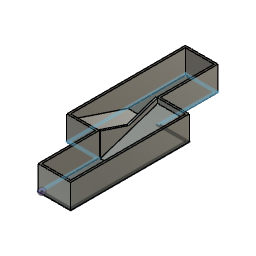
SandGravelMulch v1 (Autodesk Fusion 360 design; units mm, degrees)
Autodesk Fusion 360 part; units mm, degrees
sketch "Sketch1" plane through (0, 0, 0) normal (0, 0, 1) x (1, 0, 0)
  line L0 (0, 0) -> (300, 0)
  line L1 (300, 0) -> (300, 1200)
  line L2 (300, 1200) -> (0, 1200)
  line L3 (0, 600) -> (-300, 600)
  line L4 (-300, 600) -> (-300, 1800)
  line L5 (-300, 1800) -> (0, 1800)
  line L6 (0, 1800) -> (0, 1200)
  line L7 (0, 0) -> (0, 600)
  line L8 (20, 1820) -> (20, 1220)
  line L9 (320, 1220) -> (20, 1220)
  line L10 (320, -20) -> (320, 1220)
  line L11 (-20, -20) -> (320, -20)
  line L12 (-20, -20) -> (-20, 580)
  line L13 (-20, 580) -> (-320, 580)
  line L14 (-320, 580) -> (-320, 1820)
  line L15 (-320, 1820) -> (20, 1820)
  dimension "d1" = 300
  dimension "d2" = 1200
  dimension "d3" = 300
  dimension "d4" = 1200
  dimension "d5" = -20
  constraint horizontal L0
  constraint vertical L1
  constraint horizontal L2
  constraint coincident L0.start L7.start
  constraint perpendicular L3 L4
  constraint perpendicular L4 L5
  constraint perpendicular L2 L6
  constraint perpendicular L3 L7
  measures "d1" distance of L0.start L0.end
  measures "d2" distance of L0.end L1.end
  measures "d3" distance of L3.start L3.end
  measures "d4" distance of L3.end L4.end
extrude "Extrude1" add sketch "Sketch1" along normal blind 400 makes body 1
extrude "Extrude2" add sketch "Sketch1" against normal blind 5 separate body contours L0 L1 L2 L3 L4 L5 L6 L7 makes body 2
extrude "Extrude3" add sketch "Sketch1" against normal blind 5 bodies 1 2
extrude "Extrude4" cut 1 faces at (-313.3333, 1400, 400) along direction (0, 0, -1) blind 100 on bodies 1 bodies 1
extrude "Extrude5" cut 1 faces at (-313.3333, 1400, 300) along direction (0, 0, -1) blind 50 on bodies 1 bodies 1
sketch "Sketch2" plane through (300, 0, 0) normal (-1, 0, 0) x (0, -1, 0)
  line L0 (0, 250) -> (-1200, 250)
  line L1 (-1200, 250) -> (-1200, 0)
  line L2 (-1200, 0) -> (0, 0)
  line L3 (0, 0) -> (0, 250)
  line L4 (-600, 250) -> (-600, 0) construction
  line L5 (-1200, 250) -> (-1200, 200) construction
  line L6 (-1200, 200) -> (-600, 0)
  dimension "d16" = 50
  constraint midpoint L0 L4.start
  constraint midpoint L2 L4.end
  constraint coincident L0.end L1.start
  constraint perpendicular L0 L5
  measures "d16" distance of L0.end L5.end
extrude "Extrude6" add sketch "Sketch2" along normal blind 300 contours L1 L2 L6 bodies 1
sketch "Sketch3" plane through (-300, 0, 0) normal (1, 0, 0) x (0, 1, 0)
  line L0 (1800, 250) -> (600, 250)
  line L1 (600, 250) -> (600, 0)
  line L2 (600, 0) -> (1800, 0)
  line L3 (1800, 0) -> (1800, 250)
  line L4 (1200, 250) -> (1200, 0) construction
  line L5 (600, 250) -> (600, 200) construction
  line L6 (600, 200) -> (1200, 0)
  dimension "d19" = 50
  constraint midpoint L0 L4.start
  constraint midpoint L2 L4.end
  constraint coincident L0.end L1.start
  constraint perpendicular L0 L5
  measures "d19" distance of L0.end L5.end
extrude "Extrude7" add sketch "Sketch3" along normal blind 300 contours L1 L2 L6 bodies 1
sketch "Sketch4" plane through (0, 0, 0) normal (-1, 0, 0) x (0, -1, 0)
  line L0 (-1200, 0) -> (-900, 100)
  line L1 (-900, 100) -> (-1200, 200)
  line L2 (-1200, 200) -> (-1200, 250)
  line L3 (-1200, 250) -> (-1800, 250)
  line L4 (-1800, 250) -> (-1800, 0)
  line L5 (-1800, 0) -> (-1200, 0)
  line L6 (-900, 100) -> (-900, 150)
  line L7 (-1200, 250) -> (-900, 150)
  dimension "d22" = 50
  constraint coincident L0.end L1.start
  constraint vertical L6
  constraint coincident L2.end L3.start
  measures "d22" distance of L0.end L6.end
sketch "Sketch5" plane through (0, 0, 0) normal (1, 0, 0) x (0, 1, 0)
  line L0 (600, 250) -> (0, 250)
  line L1 (0, 250) -> (0, 0)
  line L2 (0, 0) -> (600, 0)
  line L3 (600, 0) -> (900, 100)
  line L4 (900, 100) -> (600, 200)
  line L5 (600, 200) -> (600, 250)
  line L6 (900, 100) -> (900, 150)
  line L7 (900, 150) -> (600, 250)
  dimension "d23" = 50
  constraint coincident L3.end L4.start
  constraint vertical L6
  constraint coincident L0.start L5.end
  measures "d23" distance of L3.end L6.end
extrude "Extrude8" add sketch "Sketch5" sketch "Sketch4" against normal mid plane 20 contours L4 L5 L6 L7 of sketch 2 contours L1 L2 L6 L7 bodies 1
sketch "Sketch6" plane through (0, 0, 0) normal (-1, 0, 0) x (0, -1, 0)
  line L0 (-1200, 0) -> (-900, 100)
  line L1 (-900, 100) -> (-1200, 200)
  line L2 (-1200, 200) -> (-1200, 250)
  line L3 (-1200, 250) -> (-1800, 250)
  line L4 (-1800, 250) -> (-1800, 0)
  line L5 (-1800, 0) -> (-1200, 0)
  line L6 (-1200, 0) -> (-1200, 200)
  constraint coincident L0.start L5.end
  constraint coincident L1.end L2.start
extrude "Extrude9" add sketch "Sketch6" along normal blind 10 contours L0 L1 L6 bodies 1
sketch "Sketch7" plane through (0, 0, 0) normal (1, 0, 0) x (0, 1, 0)
  line L0 (600, 250) -> (0, 250)
  line L1 (0, 250) -> (0, 0)
  line L2 (0, 0) -> (600, 0)
  line L3 (600, 0) -> (900, 100)
  line L4 (900, 100) -> (600, 200)
  line L5 (600, 200) -> (600, 250)
  line L6 (600, 200) -> (600, 0)
  constraint coincident L4.end L5.start
  constraint coincident L2.end L3.start
extrude "Extrude10" add sketch "Sketch7" along normal blind 10 contours L3 L4 L6 bodies 1
